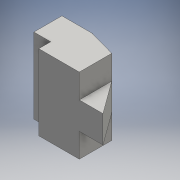
# Autodesk Inventor part: 240628_final1
Saved by Autodesk Inventor 2016 (Build 200138000, 138)
## iProperties
Created: 2024-06-28
Part Number: 240628_final1
Material: 일반
Document SubType Name: Modeling
Designer: pc
Density: 1 g/cm^3
Appearance: 기본값
Author: pc
Autodesk Inventor part; units mm, degrees
ref_plane "YZ Plane" through (0, 0, 0) normal (1, 0, 0) x (0, 1, 0)
ref_plane "XZ Plane" through (0, 0, 0) normal (0, 1, 0) x (-1, 0, 0)
ref_plane "XY Plane" through (0, 0, 0) normal (0, 0, 1) x (1, 0, 0)
sketch "스케치1" plane through (0, 0, 0) normal (0, 0, 1) x (1, 0, 0)
  line L0 (26.8403, -18.2471) -> (-26.8403, -18.2471)
  line L1 (-26.8403, -18.2471) -> (-26.8403, 18.2471)
  line L2 (-26.8403, 18.2471) -> (26.8403, 18.2471)
  line L3 (26.8403, 18.2471) -> (26.8403, -18.2471)
  line L4 (26.8403, -18.2471) -> (-26.8403, 18.2471) construction
  line L5 (-26.8403, -18.2471) -> (26.8403, 18.2471) construction
  point P0 (0, 0)
  constraints: 12 end point, 2 midpoint, 2 parallel, 1 horizontal, 1 perpendicular
extrude "돌출1" add sketch "스케치1" along normal blind 50
sketch "스케치2" plane through (-26.8403, 18.2471, 0) normal (0, 1, 0) x (1, 0, 0)
  line L0 (0, -50) -> (53.6805, -50) projected
  line L1 (0, -50) -> (20, -50)
  line L2 (20, -50) -> (20, -34)
  line L3 (20, -34) -> (0, -34)
  line L4 (0, -34) -> (0, -50)
  line L5 (0, 0) -> (20, 0)
  line L6 (20, 0) -> (20, -16)
  line L7 (20, -16) -> (0, -16)
  line L8 (0, -16) -> (0, 0)
  line L9 (20, -34) -> (38, -34)
  line L10 (38, -34) -> (38, -16)
  line L11 (38, -16) -> (20, -16)
  line L12 (20, -16) -> (20, -34)
  line L13 (38, -34) -> (53.6805, -34)
  line L14 (53.6805, -34) -> (53.6805, -50)
  line L15 (53.6805, -50) -> (38, -50)
  line L16 (38, -50) -> (38, -34)
  line L17 (53.6805, 0) -> (53.6805, -50) projected
  line L18 (38, -16) -> (53.6805, -16)
  line L19 (53.6805, -16) -> (53.6805, 0)
  line L20 (53.6805, 0) -> (38, 0)
  line L21 (38, 0) -> (38, -16)
  point P0 (26.8403, 0)
  dimension "d2" = 20
  dimension "d3" = 16
  dimension "d4" = 20
  dimension "d5" = 16
  dimension "d6" = 18
  constraints: 40 end point, 10 parallel, 5 horizontal, 5 perpendicular, 2 point on line
  measures "d2" distance of L3.end L2.end
  measures "d3" distance of L2.end L1.end
  measures "d4" distance of L6.end L7.end
  measures "d5" distance of L5.end L6.end
  measures "d6" distance of L11.end L10.end
extrude "돌출2" cut sketch "스케치2" against normal blind 10 contours L4 L3 L2 L0 | L7 L8 L5 L6
extrude "돌출3" cut sketch "스케치2" against normal blind 15 contours L12 L11 L10 L9
extrude "돌출4" cut sketch "스케치2" against normal blind 50 contours L16 L13 L14 L0 | L21 L20 L17 L18
sketch "스케치3" plane through (11.1597, 18.2471, 34) normal (0, 0, 1) x (1, 0, 0)
  line L0 (15.6805, -36.4941) -> (15.6805, 0) projected
  line L1 (0, -15) -> (15.6805, -36.4941)
  line L2 (15.6805, -36.4941) -> (15.6805, 0)
  line L3 (0, -36.4941) -> (0, 0) projected
  line L4 (15.6805, 0) -> (0, 0)
  line L5 (0, 0) -> (0, -15)
  point P0 (-11.1597, -18.2471)
  constraints: 8 end point, 2 perpendicular, 1 collinear
extrude "돌출5" cut sketch "스케치3" against normal blind 50
sketch "스케치4" plane through (0, 0, 50) normal (0, 0, 1) x (1, 0, 0)
  line L0 (-6.8403, 8.2471) -> (-6.8403, 18.2471) projected
  line L1 (-6.8403, 3.2471) -> (11.1597, 3.2471) projected
  line L2 (-6.8403, 8.2471) -> (11.1597, 3.2471)
  line L3 (11.1597, 18.2471) -> (-6.8403, 18.2471) projected
  line L4 (11.1597, 3.2471) -> (11.1597, 18.2471)
  line L5 (11.1597, 18.2471) -> (-6.8403, 18.2471)
  line L6 (-6.8403, 18.2471) -> (-6.8403, 8.2471)
  point P0 (0, 0)
  constraints: 8 end point, 2 perpendicular, 1 collinear
extrude "돌출6" cut sketch "스케치4" against normal blind 50
sketch "스케치5" plane through (0, 0, 50) normal (0, 0, 1) x (1, 0, 0)
  line L0 (-26.8403, 8.2471) -> (-26.8403, -18.2471) projected
  line L1 (-26.8403, -18.2471) -> (11.1597, -18.2471) projected
  line L2 (-26.8403, -10.3165) -> (-15.6784, -10.3165)
  line L3 (-15.6784, -10.3165) -> (-15.6784, -18.2471)
  line L4 (-15.6784, -18.2471) -> (-26.8403, -18.2471)
  line L5 (-26.8403, -18.2471) -> (-26.8403, -10.3165)
  point P0 (0, 0)
  constraints: 8 end point, 2 parallel, 2 point on line, 1 horizontal, 1 perpendicular
extrude "돌출7" cut sketch "스케치5" against normal blind 50
